Spike Norbert (Autodesk Fusion 360 design; units mm, degrees)
Autodesk Fusion 360 part; units mm, degrees
sketch "Sketch1" plane through (0, 0, 0) normal (0, 0, 1) x (1, 0, 0)
  circle A0 centre (0, 0) radius 2
  circle A1 centre (0, 0) radius 4
  circle A2 centre (0, 0) radius 1
  dimension "d1" = 4
  dimension "d2" = 8
  dimension "d8" = 2
  constraint coincident A0.centre A1.centre
  constraint concentric A0 A2
  measures "d1" diameter of A0
  measures "d2" diameter of A1
  measures "d8" diameter of A2
extrude "Extrude4" add sketch "Sketch1" along normal blind 5 contours A0 | A2
sketch "Sketch2" plane through (0, 0, 5) normal (0, 0, 1) x (-1, 0, 0)
  circle A0 centre (0, 0) radius 2
  circle A1 centre (0, 0) radius 4
  dimension "d13" = 8
  constraint coincident A0.centre A1.centre
  measures "d13" diameter of A1
sketch "Sketch3" plane through (0, 0, 5) normal (0, 0, 1) x (1, 0, 0)
sketch "Sketch4" plane through (0, 0, 5) normal (0, 0, 1) x (1, 0, 0)
ref_plane "WorkPlane1" through (0, 0, 15) normal (0, 0, 1) x (-1, 0, 0)
sketch "Sketch5" plane through (0, 0, 15) normal (0, 0, 1) x (1, 0, 0)
  circle A0 centre (0, 0) radius 1
  dimension "d16" = 2
  constraint coincident A0.centre origin
  measures "d16" diameter of A0
loft "Loft1" add profiles "Sketch5", "Sketch2" section 1 section 2
